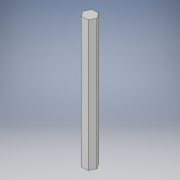
# Autodesk Inventor part: hex shaft
Saved by Autodesk Inventor 2018 (Build 220112000, 112)
## iProperties
Created: 2019-01-23
Part Number: hex shaft
Material: Generic
Document SubType Name: Modeling
Designer: s-2513225
Density: 1 g/cm^3
Appearance: Default
Author: s-2513225
Autodesk Inventor part; units mm, degrees
ref_plane "YZ Plane" through (0, 0, 0) normal (1, 0, 0) x (0, 1, 0)
ref_plane "XZ Plane" through (0, 0, 0) normal (0, 1, 0) x (-1, 0, 0)
ref_plane "XY Plane" through (0, 0, 0) normal (0, 0, 1) x (1, 0, 0)
sketch "Sketch1" plane through (0, 0, 0) normal (0, 1, 0) x (-1, 0, 0)
  line L0 (3.5713, -5.2505) -> (-2.7614, -5.7181)
  line L1 (-2.7614, -5.7181) -> (-6.3328, -0.4676)
  line L2 (-6.3328, -0.4676) -> (-3.5713, 5.2505)
  line L3 (-3.5713, 5.2505) -> (2.7614, 5.7181)
  line L4 (2.7614, 5.7181) -> (6.3328, 0.4676)
  line L5 (6.3328, 0.4676) -> (3.5713, -5.2505)
  line L6 (3.5713, -5.2505) -> (-3.5713, 5.2505) construction
  point P0 (0, 0)
  point P1 (0, 0)
  dimension "d1" = 12.7
  constraints: 14 end point, 1 coincident, 13 other
  measures "d1" distance of L0.start L2.end
extrude "Extrusion1" add sketch "Sketch1" along normal blind 127
body "Solid1"
